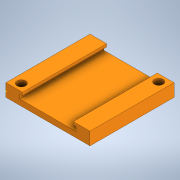
# Autodesk Inventor part: rplidar_adapter_board_holder
Saved by Autodesk Inventor 2020.3 (Build 243373000, 373)
## iProperties
Created: 2020-07-04
Part Number: rplidar_adapter_board_holder
Material: PET Plastic
Document SubType Name: Modeling
Designer: Devin
Density: 1.541 g/cm^3
Appearance: Orange
Author: Devin
Autodesk Inventor part; units mm, degrees
ref_plane "YZ Plane" through (0, 0, 0) normal (1, 0, 0) x (0, 1, 0)
ref_plane "XZ Plane" through (0, 0, 0) normal (0, 1, 0) x (-1, 0, 0)
ref_plane "XY Plane" through (0, 0, 0) normal (0, 0, 1) x (1, 0, 0)
sketch "Sketch1" plane through (0, 0, 0) normal (0, 1, 0) x (-1, 0, 0)
  line L0 (0, 0) -> (0, -30)
  line L1 (0, -30) -> (-30, -30)
  line L2 (-30, -30) -> (-30, 0)
  line L3 (-30, 0) -> (0, 0)
  dimension "d0" = 30
  dimension "d1" = 30
  constraints: 8 end point, 2 parallel, 1 perpendicular, 1 vertical
  measures "d0" distance of L0.start L0.end
  measures "d1" distance of L0.end L1.end
extrude "Extrusion1" add sketch "Sketch1" along normal blind 2
sketch "Sketch2" plane through (0, 2, 0) normal (0, 1, 0) x (1, 0, 0)
  line L0 (0, 30) -> (0, 0) projected
  line L1 (25.05, 0) -> (30, 0)
  line L2 (30, 0) -> (30, 30) projected
  line L3 (30, 0) -> (30, 30)
  line L4 (30, 30) -> (25.05, 30)
  line L5 (25.05, 30) -> (25.05, 0)
  line L6 (30, 0) -> (30, 30)
  line L7 (0, 0) -> (30, 0) projected
  line L8 (30, 30) -> (0, 30) projected
  line L9 (4.95, 0) -> (0, 0)
  line L10 (0, 0) -> (0, 30)
  line L11 (0, 30) -> (4.95, 30)
  line L12 (4.95, 30) -> (4.95, 0)
  point P0 (4.95, 0)
  constraints: 18 end point, 2 collinear
extrude "Extrusion2" add sketch "Sketch2" along normal blind 1.56 contours L8 L12 L7 L0 | L4 L2 L1 L5
sketch "Sketch3" plane through (0, 3.56, 0) normal (0, 1, 0) x (1, 0, 0)
  line L0 (0, 30) -> (0, 0) projected
  line L1 (0, 0) -> (0, 30)
  line L2 (0, 30) -> (5.95, 30)
  line L3 (5.95, 30) -> (5.95, 0)
  line L4 (5.95, 0) -> (0, 0)
  line L5 (4.95, 0) -> (25.05, 0) projected
  line L6 (25.05, 30) -> (4.95, 30) projected
  line L7 (30, 30) -> (30, 0)
  line L8 (30, 0) -> (30, 30)
  line L9 (30, 30) -> (24.05, 30)
  line L10 (24.05, 30) -> (24.05, 0)
  line L11 (24.05, 0) -> (30, 0)
  point P0 (24.05, 0)
  dimension "d8" = 30
  dimension "d9" = 5.95
  constraints: 18 end point, 2 parallel, 1 perpendicular, 1 vertical
  measures "d8" distance of L0.start L0.end
  measures "d9" distance of L3.end L0.end
extrude "Extrusion3" add sketch "Sketch3" along normal blind 1 contours L2 L3 L4 L0 | L6 L9 L7 L11 L5 L10
sketch "Sketch5" plane through (0, 4.56, 0) normal (0, 1, 0) x (1, 0, 0)
  circle A0 centre (2.975, 2.5) radius 1.55
  circle A1 centre (27.025, 27.5) radius 1.55
  line L0 (30, 30) -> (24.05, 30) projected
  line L1 (30, 0) -> (30, 30) projected
  line L2 (0, 30) -> (0, 0) projected
  line L3 (0, 0) -> (5.95, 0) projected
  dimension "d13" = 3.1
  dimension "d14" = 3.1
  dimension "d15" = 2.5
  dimension "d16" = 2.975
  dimension "d18" = 2.975
  dimension "d19" = 2.5
  constraints: 2 centre point
  measures "d13" diameter of A0
  measures "d14" diameter of A1
  measures "d15" distance from line of L0 A1.centre
  measures "d16" distance from line of L1 A1.centre
  measures "d18" distance from line of L2 A0.centre
  measures "d19" distance from line of L3 A0.centre
extrude "Extrusion4" cut sketch "Sketch5" against normal blind 10
sketch "Sketch6" plane through (0, 2, 0) normal (0, 1, 0) x (1, 0, 0)
  circle A0 centre (27.025, 27.5) radius 1.55 projected
  point P0 (0, 0)
body "Solid1"
